Autodesk Inventor part; units mm, degrees
note: some values were not read from the file. Chosen so that the rebuilt part matches the saved one: direction of "Hole1"; direction of "Hole2"; direction of "Hole4"; direction of "Hole6"; direction of "Hole7".
(part 2 of 2)
sketch "Sketch15" plane through (90, 0, 36) normal (1, 0, 0) x (0, 0, -1)
  line L0 (36.5, 36.75) -> (45.5, 36.75) construction
  line L1 (45.5, 36.75) -> (45.5, 33.25) construction
  line L2 (45.5, 33.25) -> (36.5, 33.25) construction
  line L3 (36.5, 33.25) -> (36.5, 36.75) construction
  line L4 (54.5, 21.75) -> (63.5, 21.75) construction
  line L5 (63.5, 21.75) -> (63.5, 18.25) construction
  line L6 (63.5, 18.25) -> (54.5, 18.25) construction
  line L7 (54.5, 18.25) -> (54.5, 21.75) construction
  line L8 (36.5, 21.75) -> (45.5, 21.75) construction
  line L9 (45.5, 21.75) -> (45.5, 18.25) construction
  line L10 (45.5, 18.25) -> (36.5, 18.25) construction
  line L11 (36.5, 18.25) -> (36.5, 21.75) construction
  line L12 (54.5, 36.75) -> (63.5, 36.75) construction
  line L13 (63.5, 36.75) -> (63.5, 33.25) construction
  line L14 (63.5, 33.25) -> (54.5, 33.25) construction
  line L15 (54.5, 33.25) -> (54.5, 36.75) construction
  circle A0 centre (24.5, 15.5) radius 1.75 construction
  circle A1 centre (15, 27.5) radius 12 construction
  circle A2 centre (50, 20) radius 3.25 construction
  circle A3 centre (5.5, 39.5) radius 1.75 construction
  circle A4 centre (50, 35) radius 3.25 construction
  line L16 (0, 0) -> (72, 0) construction
  line L17 (72, 0) -> (72, 48) construction
  line L18 (0, 48) -> (72, 48) construction
  line L19 (0, 0) -> (0, 48) construction
  spline S0 degree 2 poles (39.3099, 33.653) (39.3099, 33.468) (39.1295, 33.468) knots 0 0 0 1 1 1
  spline S1 degree 2 poles (39.1295, 33.468) (38.9468, 33.468) (38.9468, 33.6554) knots 0 0 0 1 1 1
  line L20 (38.9468, 33.6554) -> (38.9468, 35.8082)
  line L21 (38.9468, 35.8082) -> (38.2838, 34.8477)
  spline S2 degree 2 poles (38.2838, 34.8477) (38.1971, 34.7189) (38.073, 34.7189) knots 0 0 0 1 1 1
  spline S3 degree 2 poles (38.073, 34.7189) (37.9512, 34.7189) (37.8762, 34.8337) knots 0 0 0 1 1 1
  line L22 (37.8762, 34.8337) -> (37.2203, 35.8316)
  line L23 (37.2203, 35.8316) -> (37.2203, 33.6554)
  spline S4 degree 2 poles (37.2203, 33.6554) (37.2203, 33.468) (37.0376, 33.468) knots 0 0 0 1 1 1
  spline S5 degree 2 poles (37.0376, 33.468) (36.8525, 33.468) (36.8525, 33.6554) knots 0 0 0 1 1 1
  line L24 (36.8525, 33.6554) -> (36.8525, 36.2978)
  spline S6 degree 2 poles (36.8525, 36.2978) (36.8525, 36.4969) (37.0516, 36.4969) knots 0 0 0 1 1 1
  spline S7 degree 2 poles (37.0516, 36.4969) (37.1992, 36.4969) (37.2953, 36.3587) knots 0 0 0 1 1 1
  line L25 (37.2953, 36.3587) -> (38.08, 35.2249)
  line L26 (38.08, 35.2249) -> (38.8671, 36.354)
  spline S8 degree 2 poles (38.8671, 36.354) (38.9819, 36.518) (39.1201, 36.518) knots 0 0 0 1 1 1
  spline S9 degree 2 poles (39.1201, 36.518) (39.1998, 36.518) (39.3099, 36.3938) (39.3099, 36.2954) knots 0 0 0 1 2 2 2
  line L27 (39.3099, 36.2954) -> (39.3099, 33.653)
  spline S10 degree 2 poles (42.3716, 33.7116) (42.3833, 33.6718) (42.3833, 33.6366) knots 0 0 0 1 1 1
  spline S11 degree 2 poles (42.3833, 33.6366) (42.3833, 33.5617) (42.2685, 33.4633) (42.1982, 33.4633) knots 0 0 0 1 2 2 2
  spline S12 degree 2 poles (42.1982, 33.4633) (42.0717, 33.4633) (42.0272, 33.5781) knots 0 0 0 1 1 1
  line L28 (42.0272, 33.5781) -> (41.8515, 34.0302)
  line L29 (41.8515, 34.0302) -> (40.4015, 34.0302)
  line L30 (40.4015, 34.0302) -> (40.2281, 33.5781)
  spline S13 degree 2 poles (40.2281, 33.5781) (40.1836, 33.4633) (40.0642, 33.4633) knots 0 0 0 1 1 1
  spline S14 degree 2 poles (40.0642, 33.4633) (39.9892, 33.4633) (39.8744, 33.564) (39.8744, 33.6366) knots 0 0 0 1 2 2 2
  spline S15 degree 2 poles (39.8744, 33.6366) (39.8744, 33.6718) (39.8885, 33.7116) knots 0 0 0 1 1 1
  line L31 (39.8885, 33.7116) -> (40.8887, 36.3938)
  spline S16 degree 2 poles (40.8887, 36.3938) (40.9426, 36.5367) (41.1066, 36.5367) knots 0 0 0 1 1 1
  spline S17 degree 2 poles (41.1066, 36.5367) (41.2752, 36.5367) (41.3291, 36.3938) knots 0 0 0 1 1 1
  line L32 (41.3291, 36.3938) -> (42.3716, 33.7116)
  line L33 (41.7133, 34.4026) -> (41.1066, 35.9534)
  line L34 (41.1066, 35.9534) -> (40.542, 34.4026)
  line L35 (40.542, 34.4026) -> (41.7133, 34.4026)
  spline S18 degree 2 poles (45.0022, 33.6507) (45.0022, 33.4633) (44.8547, 33.4633) knots 0 0 0 1 1 1
  spline S19 degree 2 poles (44.8547, 33.4633) (44.7422, 33.4633) (44.6532, 33.5898) knots 0 0 0 1 1 1
  line L36 (44.6532, 33.5898) -> (43.161, 35.7684)
  line L37 (43.161, 35.7684) -> (43.161, 33.653)
  spline S20 degree 2 poles (43.161, 33.653) (43.161, 33.4633) (42.9806, 33.4633) knots 0 0 0 1 1 1
  spline S21 degree 2 poles (42.9806, 33.4633) (42.7979, 33.4633) (42.7979, 33.653) knots 0 0 0 1 1 1
  line L38 (42.7979, 33.653) -> (42.7979, 36.3399)
  spline S22 degree 2 poles (42.7979, 36.3399) (42.7979, 36.518) (42.9619, 36.518) knots 0 0 0 1 1 1
  spline S23 degree 2 poles (42.9619, 36.518) (43.0767, 36.518) (43.161, 36.3985) knots 0 0 0 1 1 1
  line L39 (43.161, 36.3985) -> (44.6392, 34.2574)
  line L40 (44.6392, 34.2574) -> (44.6392, 36.3259)
  spline S24 degree 2 poles (44.6392, 36.3259) (44.6392, 36.518) (44.8219, 36.518) knots 0 0 0 1 1 1
  spline S25 degree 2 poles (44.8219, 36.518) (45.0022, 36.518) (45.0022, 36.3259) knots 0 0 0 1 1 1
  line L41 (45.0022, 36.3259) -> (45.0022, 33.6507)
  spline S26 degree 2 poles (57.133, 35.6395) (57.133, 35.178) (56.8308, 34.9461) knots 0 0 0 1 1 1
  spline S27 degree 2 poles (56.8308, 34.9461) (56.6317, 34.7962) (56.4326, 34.7962) knots 0 0 0 1 1 1
  line L42 (56.4326, 34.7962) -> (56.3881, 34.7939)
  line L43 (56.3881, 34.7939) -> (57.0978, 33.7772)
  spline S28 degree 2 poles (57.0978, 33.7772) (57.133, 33.7233) (57.133, 33.6647) knots 0 0 0 1 1 1
  spline S29 degree 2 poles (57.133, 33.6647) (57.133, 33.5898) (57.0182, 33.475) (56.9479, 33.475) knots 0 0 0 1 2 2 2
  spline S30 degree 2 poles (56.9479, 33.475) (56.8636, 33.475) (56.8097, 33.5546) knots 0 0 0 1 1 1
  line L44 (56.8097, 33.5546) -> (55.9359, 34.7962)
  line L45 (55.9359, 34.7962) -> (55.355, 34.7962)
  line L46 (55.355, 34.7962) -> (55.355, 33.6647)
  spline S31 degree 2 poles (55.355, 33.6647) (55.355, 33.475) (55.1746, 33.475) knots 0 0 0 1 1 1
  spline S32 degree 2 poles (55.1746, 33.475) (54.9919, 33.475) (54.9919, 33.6647) knots 0 0 0 1 1 1
  line L47 (54.9919, 33.6647) -> (54.9919, 36.5133)
  line L48 (54.9919, 36.5133) -> (56.2733, 36.5133)
  spline S33 degree 2 poles (56.2733, 36.5133) (56.6223, 36.5133) (56.8706, 36.2861) knots 0 0 0 1 1 1
  spline S34 degree 2 poles (56.8706, 36.2861) (57.133, 36.0377) (57.133, 35.6395) knots 0 0 0 1 1 1
  spline S35 degree 2 poles (56.7746, 35.6395) (56.7746, 35.8738) (56.6247, 36.0167) knots 0 0 0 1 1 1
  spline S36 degree 2 poles (56.6247, 36.0167) (56.4818, 36.1455) (56.2733, 36.1455) knots 0 0 0 1 1 1
  line L49 (56.2733, 36.1455) -> (55.355, 36.1455)
  line L50 (55.355, 36.1455) -> (55.355, 35.1687)
  line L51 (55.355, 35.1687) -> (56.4326, 35.1687)
  spline S37 degree 2 poles (56.4326, 35.1687) (56.531, 35.1687) (56.6317, 35.2624) knots 0 0 0 1 1 1
  spline S38 degree 2 poles (56.6317, 35.2624) (56.7746, 35.3912) (56.7746, 35.6395) knots 0 0 0 1 1 1
  line L52 (59.5013, 33.5148) -> (57.6882, 33.5148)
  line L53 (57.6882, 33.5148) -> (57.6882, 36.5156)
  line L54 (57.6882, 36.5156) -> (59.5013, 36.5156)
  spline S39 degree 2 poles (59.5013, 36.5156) (59.684, 36.5156) (59.684, 36.3306) knots 0 0 0 1 1 1
  spline S40 degree 2 poles (59.684, 36.3306) (59.684, 36.1432) (59.5013, 36.1432) knots 0 0 0 1 1 1
  line L55 (59.5013, 36.1432) -> (58.0466, 36.1432)
  line L56 (58.0466, 36.1432) -> (58.0466, 35.3467)
  line L57 (58.0466, 35.3467) -> (59.4123, 35.3467)
  spline S41 degree 2 poles (59.4123, 35.3467) (59.595, 35.3467) (59.595, 35.1616) knots 0 0 0 1 1 1
  spline S42 degree 2 poles (59.595, 35.1616) (59.595, 34.9742) (59.4123, 34.9742) knots 0 0 0 1 1 1
  line L58 (59.4123, 34.9742) -> (58.0466, 34.9742)
  line L59 (58.0466, 34.9742) -> (58.0466, 33.8873)
  line L60 (58.0466, 33.8873) -> (59.5013, 33.8873)
  spline S43 degree 2 poles (59.5013, 33.8873) (59.684, 33.8873) (59.684, 33.7022) knots 0 0 0 1 1 1
  spline S44 degree 2 poles (59.684, 33.7022) (59.684, 33.5148) (59.5013, 33.5148) knots 0 0 0 1 1 1
  spline S45 degree 2 poles (62.7926, 33.6601) (62.7926, 33.475) (62.6122, 33.475) knots 0 0 0 1 1 1
  spline S46 degree 2 poles (62.6122, 33.475) (62.4295, 33.475) (62.4295, 33.6624) knots 0 0 0 1 1 1
  line L61 (62.4295, 33.6624) -> (62.4295, 35.8152)
  line L62 (62.4295, 35.8152) -> (61.7666, 34.8548)
  spline S47 degree 2 poles (61.7666, 34.8548) (61.6799, 34.7259) (61.5557, 34.7259) knots 0 0 0 1 1 1
  spline S48 degree 2 poles (61.5557, 34.7259) (61.4339, 34.7259) (61.3589, 34.8407) knots 0 0 0 1 1 1
  line L63 (61.3589, 34.8407) -> (60.703, 35.8386)
  line L64 (60.703, 35.8386) -> (60.703, 33.6624)
  spline S49 degree 2 poles (60.703, 33.6624) (60.703, 33.475) (60.5203, 33.475) knots 0 0 0 1 1 1
  spline S50 degree 2 poles (60.5203, 33.475) (60.3353, 33.475) (60.3353, 33.6624) knots 0 0 0 1 1 1
  line L65 (60.3353, 33.6624) -> (60.3353, 36.3048)
  spline S51 degree 2 poles (60.3353, 36.3048) (60.3353, 36.5039) (60.5344, 36.5039) knots 0 0 0 1 1 1
  spline S52 degree 2 poles (60.5344, 36.5039) (60.682, 36.5039) (60.778, 36.3657) knots 0 0 0 1 1 1
  line L66 (60.778, 36.3657) -> (61.5627, 35.2319)
  line L67 (61.5627, 35.2319) -> (62.3498, 36.361)
  spline S53 degree 2 poles (62.3498, 36.361) (62.4646, 36.525) (62.6028, 36.525) knots 0 0 0 1 1 1
  spline S54 degree 2 poles (62.6028, 36.525) (62.6825, 36.525) (62.7926, 36.4008) (62.7926, 36.3025) knots 0 0 0 1 2 2 2
  line L68 (62.7926, 36.3025) -> (62.7926, 33.6601)
  line L69 (39.1962, 18.5886) -> (37.3831, 18.5886)
  line L70 (37.3831, 18.5886) -> (37.3831, 21.4044)
  spline S55 degree 2 poles (37.3831, 21.4044) (37.3831, 21.5941) (37.5635, 21.5941) knots 0 0 0 1 1 1
  spline S56 degree 2 poles (37.5635, 21.5941) (37.7415, 21.5941) (37.7415, 21.4044) knots 0 0 0 1 1 1
  line L71 (37.7415, 21.4044) -> (37.7415, 18.9564)
  line L72 (37.7415, 18.9564) -> (39.1962, 18.9564)
  spline S57 degree 2 poles (39.1962, 18.9564) (39.379, 18.9564) (39.379, 18.7737) knots 0 0 0 1 1 1
  spline S58 degree 2 poles (39.379, 18.7737) (39.379, 18.5886) (39.1962, 18.5886) knots 0 0 0 1 1 1
  spline S59 degree 2 poles (41.8293, 20.7883) (41.8293, 20.4392) (41.4615, 20.0129) (41.1195, 20.0129) knots 0 0 0 1 2 2 2
  line L73 (41.1195, 20.0129) -> (40.2551, 20.0129)
  line L74 (40.2551, 20.0129) -> (40.2551, 18.7385)
  spline S60 degree 2 poles (40.2551, 18.7385) (40.2551, 18.5488) (40.077, 18.5488) knots 0 0 0 1 1 1
  spline S61 degree 2 poles (40.077, 18.5488) (39.8967, 18.5488) (39.8967, 18.7385) knots 0 0 0 1 1 1
  line L75 (39.8967, 18.7385) -> (39.8967, 21.5941)
  line L76 (39.8967, 21.5941) -> (41.0492, 21.5941)
  spline S62 degree 2 poles (41.0492, 21.5941) (41.4474, 21.5941) (41.6465, 21.3645) knots 0 0 0 1 1 1
  spline S63 degree 2 poles (41.6465, 21.3645) (41.8293, 21.156) (41.8293, 20.7883) knots 0 0 0 1 1 1
  spline S64 degree 2 poles (41.4709, 20.7883) (41.4709, 21.2263) (41.0492, 21.2263) knots 0 0 0 1 1 1
  line L77 (41.0492, 21.2263) -> (40.2551, 21.2263)
  line L78 (40.2551, 21.2263) -> (40.2551, 20.3853)
  line L79 (40.2551, 20.3853) -> (41.1195, 20.3853)
  spline S65 degree 2 poles (41.1195, 20.3853) (41.4709, 20.3853) (41.4709, 20.7883) knots 0 0 0 1 1 1
  line L80 (44.4225, 21.2029) -> (43.6377, 21.2029)
  line L81 (43.6377, 21.2029) -> (43.6377, 18.605)
  spline S66 degree 2 poles (43.6377, 18.605) (43.6377, 18.4059) (43.448, 18.4059) knots 0 0 0 1 1 1
  spline S67 degree 2 poles (43.448, 18.4059) (43.2559, 18.4059) (43.2559, 18.605) knots 0 0 0 1 1 1
  line L82 (43.2559, 18.605) -> (43.2559, 21.2029)
  line L83 (43.2559, 21.2029) -> (42.4711, 21.2029)
  spline S68 degree 2 poles (42.4711, 21.2029) (42.2767, 21.2029) (42.2767, 21.3997) knots 0 0 0 1 1 1
  spline S69 degree 2 poles (42.2767, 21.3997) (42.2767, 21.5941) (42.4711, 21.5941) knots 0 0 0 1 1 1
  line L84 (42.4711, 21.5941) -> (44.4225, 21.5941)
  spline S70 degree 2 poles (44.4225, 21.5941) (44.6192, 21.5941) (44.6192, 21.3997) knots 0 0 0 1 1 1
  spline S71 degree 2 poles (44.6192, 21.3997) (44.6192, 21.2029) (44.4225, 21.2029) knots 0 0 0 1 1 1
  spline S72 degree 2 poles (57.4399, 19.4846) (57.4399, 18.5219) (56.4419, 18.4469) knots 0 0 0 1 1 1
  spline S73 degree 2 poles (56.4419, 18.4469) (56.025, 18.4164) (55.697, 18.6741) knots 0 0 0 1 1 1
  spline S74 degree 2 poles (55.697, 18.6741) (55.3339, 18.9623) (55.3339, 19.4589) knots 0 0 0 1 1 1
  line L85 (55.3339, 19.4589) -> (55.3339, 21.3259)
  spline S75 degree 2 poles (55.3339, 21.3259) (55.3339, 21.5156) (55.5166, 21.5156) knots 0 0 0 1 1 1
  spline S76 degree 2 poles (55.5166, 21.5156) (55.697, 21.5156) (55.697, 21.3259) knots 0 0 0 1 1 1
  line L86 (55.697, 21.3259) -> (55.697, 19.4589)
  spline S77 degree 2 poles (55.697, 19.4589) (55.697, 19.1379) (55.9313, 18.9576) knots 0 0 0 1 1 1
  spline S78 degree 2 poles (55.9313, 18.9576) (56.1397, 18.7959) (56.4162, 18.8147) knots 0 0 0 1 1 1
  spline S79 degree 2 poles (56.4162, 18.8147) (57.0815, 18.8545) (57.0815, 19.4846) knots 0 0 0 1 1 1
  line L87 (57.0815, 19.4846) -> (57.0815, 21.3259)
  spline S80 degree 2 poles (57.0815, 21.3259) (57.0815, 21.5156) (57.2618, 21.5156) knots 0 0 0 1 1 1
  spline S81 degree 2 poles (57.2618, 21.5156) (57.4399, 21.5156) (57.4399, 21.3259) knots 0 0 0 1 1 1
  line L88 (57.4399, 21.3259) -> (57.4399, 19.4846)
  spline S82 degree 2 poles (59.9862, 19.3066) (59.9862, 18.4469) (58.9133, 18.4469) knots 0 0 0 1 1 1
  spline S83 degree 2 poles (58.9133, 18.4469) (58.2691, 18.4469) (57.9224, 19.0864) knots 0 0 0 1 1 1
  spline S84 degree 2 poles (57.9224, 19.0864) (57.8967, 19.1309) (57.8967, 19.1848) knots 0 0 0 1 1 1
  spline S85 degree 2 poles (57.8967, 19.1848) (57.8967, 19.2691) (58.0208, 19.398) (58.0958, 19.398) knots 0 0 0 1 2 2 2
  spline S86 degree 2 poles (58.0958, 19.398) (58.1801, 19.398) (58.2199, 19.3043) knots 0 0 0 1 1 1
  spline S87 degree 2 poles (58.2199, 19.3043) (58.4378, 18.8194) (58.9133, 18.8194) knots 0 0 0 1 1 1
  spline S88 degree 2 poles (58.9133, 18.8194) (59.6137, 18.8194) (59.6137, 19.3019) knots 0 0 0 1 1 1
  spline S89 degree 2 poles (59.6137, 19.3019) (59.6137, 19.5502) (59.1733, 19.7329) knots 0 0 0 1 1 1
  spline S90 degree 2 poles (59.1733, 19.7329) (58.3792, 20.0656) (58.3628, 20.075) knots 0 0 0 1 1 1
  spline S91 degree 2 poles (58.3628, 20.075) (57.9224, 20.3373) (57.9224, 20.7707) knots 0 0 0 1 1 1
  spline S92 degree 2 poles (57.9224, 20.7707) (57.9224, 21.1783) (58.2199, 21.3868) knots 0 0 0 1 1 1
  spline S93 degree 2 poles (58.2199, 21.3868) (58.4589, 21.5555) (58.8501, 21.5695) knots 0 0 0 1 1 1
  spline S94 degree 2 poles (58.8501, 21.5695) (59.2085, 21.5836) (59.4755, 21.4243) knots 0 0 0 1 1 1
  spline S95 degree 2 poles (59.4755, 21.4243) (59.759, 21.2509) (59.8621, 20.9276) knots 0 0 0 1 1 1
  spline S96 degree 2 poles (59.8621, 20.9276) (59.8691, 20.8949) (59.8691, 20.8644) knots 0 0 0 1 1 1
  spline S97 degree 2 poles (59.8691, 20.8644) (59.8691, 20.7894) (59.759, 20.6957) (59.684, 20.6957) knots 0 0 0 1 2 2 2
  spline S98 degree 2 poles (59.684, 20.6957) (59.5505, 20.6957) (59.5107, 20.8246) knots 0 0 0 1 1 1
  spline S99 degree 2 poles (59.5107, 20.8246) (59.4521, 21.0073) (59.0843, 21.2158) (58.8618, 21.2064) knots 0 0 0 1 2 2 2
  spline S100 degree 2 poles (58.8618, 21.2064) (58.2808, 21.1853) (58.2808, 20.7801) knots 0 0 0 1 1 1
  spline S101 degree 2 poles (58.2808, 20.7801) (58.2808, 20.5716) (58.4893, 20.4263) knots 0 0 0 1 1 1
  spline S102 degree 2 poles (58.4893, 20.4263) (58.6369, 20.3233) (58.9789, 20.1991) knots 0 0 0 1 1 1
  spline S103 degree 2 poles (58.9789, 20.1991) (59.4849, 20.0164) (59.6583, 19.8969) knots 0 0 0 1 1 1
  spline S104 degree 2 poles (59.6583, 19.8969) (59.9862, 19.672) (59.9862, 19.3066) knots 0 0 0 1 1 1
  spline S105 degree 2 poles (62.4881, 19.3558) (62.4881, 18.5101) (61.544, 18.5101) knots 0 0 0 1 1 1
  line L89 (61.544, 18.5101) -> (60.5273, 18.5101)
  line L90 (60.5273, 18.5101) -> (60.5273, 21.5156)
  line L91 (60.5273, 21.5156) -> (61.5042, 21.5156)
  spline S106 degree 2 poles (61.5042, 21.5156) (61.9469, 21.5156) (62.2046, 21.2861) knots 0 0 0 1 1 1
  spline S107 degree 2 poles (62.2046, 21.2861) (62.4482, 21.0588) (62.4482, 20.677) knots 0 0 0 1 1 1
  spline S108 degree 2 poles (62.4482, 20.677) (62.4482, 20.3022) (62.1414, 20.0351) knots 0 0 0 1 1 1
  spline S109 degree 2 poles (62.1414, 20.0351) (62.4881, 19.8407) (62.4881, 19.3558) knots 0 0 0 1 1 1
  spline S110 degree 2 poles (62.1296, 19.3605) (62.1296, 19.8571) (61.5206, 19.8571) knots 0 0 0 1 1 1
  line L92 (61.5206, 19.8571) -> (60.8858, 19.8571)
  line L93 (60.8858, 19.8571) -> (60.8858, 18.8826)
  line L94 (60.8858, 18.8826) -> (61.544, 18.8826)
  spline S111 degree 2 poles (61.544, 18.8826) (62.1296, 18.8826) (62.1296, 19.3605) knots 0 0 0 1 1 1
  spline S112 degree 2 poles (62.0898, 20.6817) (62.0898, 20.9042) (61.7736, 21.1432) (61.5042, 21.1432) knots 0 0 0 1 2 2 2
  line L95 (61.5042, 21.1432) -> (60.8858, 21.1432)
  line L96 (60.8858, 21.1432) -> (60.8858, 20.2296)
  line L97 (60.8858, 20.2296) -> (61.5487, 20.2296)
  spline S113 degree 2 poles (61.5487, 20.2296) (62.0898, 20.2296) (62.0898, 20.6817) knots 0 0 0 1 1 1
  point P0 (36, 0)
  point P1 (45.5, 35)
  point P2 (54.5, 35)
  point P3 (45.5, 20)
  point P4 (54.5, 20)
  dimension "d163" = 4.5
  dimension "d164" = 4.5
  dimension "d165" = 4.5
  dimension "d166" = 4.5
  dimension "d167" = 9
  dimension "d168" = 9
  dimension "d169" = 9
  dimension "d170" = 9
  dimension "d171" = 3.5
  dimension "d172" = 3.5
  constraints: 8 horizontal alignment, 4 horizontal, 4 midpoint, 8 other
  measures "d163" distance of point (45.5, 35) A4.centre
  measures "d164" distance of A4.centre point (54.5, 35)
  measures "d165" distance of A2.centre point (54.5, 20)
  measures "d166" distance of point (45.5, 20) A2.centre
  measures "d167" distance of L0.start L0.end
  measures "d168" distance of L15.end L12.end
  measures "d169" distance of L11.end L8.end
  measures "d170" distance of L7.end L4.end
  measures "d171" distance of L2.end L0.start
  measures "d172" distance of L11.start L11.end
emboss "Emboss3" sketch "Sketch15" operation cut depth 1 direction (-1, 0, 0)
sketch "Sketch16" plane through (0, 48, 0) normal (0, 1, 0) x (1, 0, 0)
  line L0 (-90, 69) -> (-94, 65) construction
  line L1 (-94, 65) -> (-94, 40) construction
  line L2 (-94, 40) -> (-90, 36) construction
  line L3 (-90, 36) -> (-90, -36) construction
  line L4 (-90, -36) -> (-94, -40) construction
  line L5 (-94, -40) -> (-94, -65) construction
  line L6 (-94, -65) -> (-90, -69) construction
  line L7 (-90, -69) -> (-65, -69) construction
  line L8 (-65, -69) -> (-61, -65) construction
  line L9 (-61, -65) -> (61, -65) construction
  line L10 (61, -65) -> (65, -69) construction
  line L11 (65, -69) -> (90, -69) construction
  line L12 (90, -69) -> (94, -65) construction
  line L13 (94, -65) -> (94, -40) construction
  line L14 (94, -40) -> (90, -36) construction
  line L15 (90, -36) -> (90, 36) construction
  line L16 (90, 36) -> (94, 40) construction
  line L17 (94, 40) -> (94, 65) construction
  line L18 (94, 65) -> (90, 69) construction
  line L19 (90, 69) -> (65, 69) construction
  line L20 (65, 69) -> (61, 65) construction
  line L21 (61, 65) -> (-61, 65) construction
  line L22 (-61, 65) -> (-65, 69) construction
  line L23 (-65, 69) -> (-90, 69) construction
  line L24 (-83, 62) -> (83, 62) construction
  line L25 (83, 62) -> (87, 58) construction
  line L26 (87, 58) -> (87, -58) construction
  line L27 (87, -58) -> (83, -62) construction
  line L28 (83, -62) -> (-83, -62) construction
  line L29 (-83, -62) -> (-87, -58) construction
  line L30 (-87, -58) -> (-87, 58) construction
  line L31 (-87, 58) -> (-83, 62) construction
  line L32 (-90, 69) -> (-87, 58) construction
  line L33 (-87, 58) -> (-83, 62) construction
  line L34 (-83, 62) -> (-94, 65) construction
  line L35 (0, 96.6) -> (0, -96.6) construction
  line L36 (-131.6, 0) -> (131.6, 0) construction
  point P0 (0, 0)
  point P1 (88.5, 63.5)
  point P2 (88.5, -63.5)
  point P3 (-88.5, -63.5)
  point P4 (-88.5, 63.5)
  constraints: 4 end point, 3 symmetric about line, 1 midpoint
hole "Hole8" at (88.5, 48, -63.5) at (88.5, 48, 63.5) at (-88.5, 48, 63.5) at (-88.5, 48, -63.5) direction (0, -1, 0) diameter 4 depth 5
equation "\"d9\" = d8"
equation "\"d10\" = d8"
equation "\"d11\" = d10"
equation "\"d12\" = d8"
equation "\"d13\" = d12"
equation "\"d14\" = d8"
equation "\"d15\" = d14"
equation "\"d77\" = d76"
equation "\"d88\" = 0.5 * d85"
equation "\"d149\" = d148"
equation "\"d154\" = d153"
equation "\"d157\" = d156"
equation "\"d159\" = d158"
equation "\"d164\" = d163"
equation "\"d165\" = d164"
equation "\"d166\" = d163"
equation "\"d168\" = d167"
equation "\"d169\" = d167"
equation "\"d170\" = d167"
body "Solid1"
